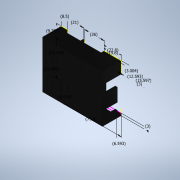
# Autodesk Inventor part: UNO Case
Saved by Autodesk Inventor 2020.1 (Build 241239000, 239)
## iProperties
Created: 2016-11-21
Part Number: UNO Case
Material: Generic
Document SubType Name: Modeling
Designer: Dimitris
Density: 1 g/cm^3
Appearance: Glossy - Black
Author: Dimitris
Autodesk Inventor part; units mm, degrees
ref_plane "YZ Plane" through (0, 0, 0) normal (1, 0, 0) x (0, 1, 0)
ref_plane "XZ Plane" through (0, 0, 0) normal (0, 1, 0) x (-1, 0, 0)
ref_plane "XY Plane" through (0, 0, 0) normal (0, 0, 1) x (1, 0, 0)
ref_plane "Work Plane2" through (0, 0, 0) normal (0, -1, 0) x (1, 0, 0)
sketch "Sketch33" plane through (0, 0, 0) normal (0, -1, 0) x (1, 0, 0)
  line L0 (74.8, -53.4338) -> (0, -53.4338)
  line L1 (0, -53.4338) -> (0, 0)
  line L2 (0, 0) -> (74.8, 0)
  line L3 (74.8, 0) -> (74.8, -53.4338)
  line L4 (74.8, -53.4338) -> (0, -53.4338)
  line L5 (0, -53.4338) -> (0, 0)
  line L6 (0, 0) -> (74.8, 0)
  line L7 (74.8, 0) -> (74.8, -53.4338)
  circle A0 centre (52, -49.5) radius 1.5 projected
  circle A1 centre (52, -49.5) radius 1.5
  circle A2 centre (3, -47.2929) radius 1.5 projected
  circle A3 centre (3, -47.2929) radius 1.5
  circle A4 centre (3, -15.7071) radius 1.5 projected
  circle A5 centre (3, -15.7071) radius 1.5
  circle A6 centre (55, -2.5) radius 1.5 projected
  circle A7 centre (55, -2.5) radius 1.5
  line L8 (74.8, -53.4338) -> (0, -53.4338)
  line L9 (0, -53.4338) -> (0, -58.4338)
  line L10 (0, -58.4338) -> (74.8, -58.4338)
  line L11 (74.8, -58.4338) -> (74.8, -53.4338)
  line L12 (0, -58.4338) -> (-5, -58.4338)
  line L13 (-5, -58.4338) -> (-5, -53.4338)
  line L14 (-5, -53.4338) -> (0, -53.4338)
  line L15 (0, -53.4338) -> (0, -58.4338)
  line L16 (0, 0) -> (-5, 0)
  line L17 (-5, 0) -> (-5, -53.4338)
  line L18 (-5, -53.4338) -> (0, -53.4338)
  line L19 (0, -53.4338) -> (0, 0)
  line L20 (-5, 0) -> (0, 0)
  line L21 (0, 0) -> (0, 5)
  line L22 (0, 5) -> (-5, 5)
  line L23 (-5, 5) -> (-5, 0)
  line L24 (0, 5) -> (74.8, 5)
  line L25 (74.8, 5) -> (74.8, 0)
  line L26 (74.8, 0) -> (0, 0)
  line L27 (0, 0) -> (0, 5)
  line L28 (74.8, -53.4338) -> (69.8, -53.4338)
  line L29 (69.8, -53.4338) -> (69.8, 5)
  line L30 (69.8, 5) -> (74.8, 5)
  line L31 (74.8, 5) -> (74.8, -53.4338)
  point P0 (74.8, 0)
  dimension "d220" = 5
  dimension "d221" = 5
  dimension "d222" = 5
  dimension "d223" = 5
  constraints: 64 end point, 16 parallel, 8 horizontal, 8 perpendicular, 4 centre point, 4 coincident, 3 point on line
  measures "d220" distance of L9.end L8.end
  measures "d221" distance of L13.end L14.end
  measures "d222" distance of L21.end L20.end
  measures "d223" distance of L29.end L30.end
extrude "Extrusion32" add sketch "Sketch33" along normal blind 5
ref_plane "Work Plane16" through (0, 0, 0) normal (0, 1, 0) x (1, 0, 0)
sketch "Sketch38" plane through (0, 0, 0) normal (0, 1, 0) x (1, 0, 0)
  line L0 (74.8, -5) -> (-5, -5) projected
  line L1 (-5, 58.4338) -> (74.8, 58.4338) projected
  line L2 (-5, -5) -> (-2, -5)
  line L3 (-2, -5) -> (-2, 58.4338)
  line L4 (-2, 58.4338) -> (-5, 58.4338)
  line L5 (-5, 58.4338) -> (-5, -5)
  line L6 (-5, -5) -> (-5, 58.4338) projected
  line L7 (74.8, 58.4338) -> (74.8, -5) projected
  line L8 (-5, 58.4338) -> (74.8, 58.4338)
  line L9 (74.8, 58.4338) -> (74.8, 55.4338)
  line L10 (74.8, 55.4338) -> (-5, 55.4338)
  line L11 (-5, 55.4338) -> (-5, 58.4338)
  line L12 (74.8, 58.4338) -> (71.8, 58.4338)
  line L13 (71.8, 58.4338) -> (71.8, 22.8825)
  line L14 (71.8, 22.8825) -> (74.8, 22.8825)
  line L15 (74.8, 22.8825) -> (74.8, 58.4338)
  line L16 (74.8, -5) -> (71.8, -5)
  line L17 (71.8, -5) -> (71.8, 10.5966)
  line L18 (71.8, 10.5966) -> (74.8, 10.5966)
  line L19 (74.8, 10.5966) -> (74.8, -5)
  line L20 (74.8, -5) -> (-5, -5)
  line L21 (-5, -5) -> (-5, -1.9965)
  line L22 (-5, -1.9965) -> (74.8, -1.9965)
  line L23 (74.8, -1.9965) -> (74.8, -5)
  point P0 (0, 0)
  point P1 (71.8, -1.9965)
  point P2 (-2, -1.9965)
  point P3 (-2, 55.4338)
  point P4 (71.8, 55.4338)
  dimension "d231" = 3
  dimension "d232" = 3
  dimension "d233" = 3
  constraints: 40 end point, 10 parallel, 6 point on line, 5 horizontal, 5 perpendicular
  measures "d231" distance of L4.end L3.end
  measures "d232" distance of L8.end L9.end
  measures "d233" distance of L14.end L13.end
extrude "Extrusion33" add sketch "Sketch38" along normal blind 20 contours L0 L17 L22 L7 | L0 L3 L22 L17 | L22 L17 L18 L7 | L0 L5 L22 L3 | L22 L5 L10 L3 | L14 L13 L10 L7 | L10 L5 L1 L3 | L3 L1 L13 L10 | L10 L13 L1 L7
ref_plane "Work Plane11" through (71.8, 0, 1.9965) normal (0, 0, -1) x (-1, 0, 0)
sketch "Sketch45" plane through (71.8, 0, 1.9965) normal (0, 0, -1) x (-1, 0, 0)
  line L0 (47.3, 2) -> (47.3, 11) projected
  line L1 (73.8, 0) -> (0, 0) projected
  line L2 (47.3, 11) -> (45.8, 11)
  line L3 (45.8, 11) -> (45.8, 0)
  line L4 (45.8, 0) -> (47.3, 0)
  line L5 (47.3, 0) -> (47.3, 11)
  line L6 (47.3, 11) -> (45.8, 11)
  line L7 (45.8, 11) -> (45.8, 20.3018)
  line L8 (45.8, 20.3018) -> (47.3, 20.3018)
  line L9 (47.3, 20.3018) -> (47.3, 11)
  line L10 (68.3, 11) -> (47.3, 11) projected
  line L11 (47.3, 20.3018) -> (68.3, 20.3018)
  line L12 (68.3, 20.3018) -> (68.3, 11)
  line L13 (68.3, 11) -> (47.3, 11)
  line L14 (47.3, 11) -> (47.3, 20.3018)
  line L15 (45.8, 11) -> (19.8, 11)
  line L16 (19.8, 11) -> (19.8, 20.3018)
  line L17 (19.8, 20.3018) -> (45.8, 20.3018)
  line L18 (45.8, 20.3018) -> (45.8, 11)
  point P0 (71.8, 0)
  dimension "d243" = 1.5
  dimension "d244" = 26
  constraints: 32 end point, 8 parallel, 4 horizontal, 4 perpendicular, 2 point on line
  measures "d243" distance of L4.end L3.end
  measures "d244" distance of L16.end L17.end
extrude "Extrusion37" cut sketch "Sketch45" against normal blind 10 contours L9 L11 L12 L10 | L15 L16 L17 L7
ref_plane "Work Plane10" through (0, 20, 0) normal (0, 1, 0) x (1, 0, 0)
sketch "Sketch46" plane through (0, 20, 0) normal (0, 1, 0) x (1, 0, 0)
  line L0 (-2, 55.4338) -> (71.8, 55.4338) projected
  line L1 (75.7583, 22.3753) -> (69.7041, 22.3753)
  line L2 (69.7041, 22.3753) -> (69.7041, 55.4338)
  line L3 (69.7041, 55.4338) -> (75.7583, 55.4338)
  line L4 (75.7583, 55.4338) -> (75.7583, 22.3753)
  point P0 (0, 0)
  constraints: 8 end point, 2 parallel, 1 horizontal, 1 perpendicular, 1 point on line
extrude "Extrusion38" cut sketch "Sketch46" against normal blind 5
ref_plane "Work Plane14" through (0, 15, 0) normal (0, 1, 0) x (1, 0, 0)
sketch "Sketch47" plane through (0, 15, 0) normal (0, 1, 0) x (1, 0, 0)
  line L0 (70.1, 40.5) -> (70.1, 49.5) projected
  line L1 (70.1, 40.5) -> (76.1155, 40.5)
  line L2 (76.1155, 40.5) -> (76.1155, 49.5)
  line L3 (76.1155, 49.5) -> (70.1, 49.5)
  line L4 (70.1, 49.5) -> (70.1, 40.5)
  point P0 (0, 0)
  dimension "d249" = 9
  constraints: 8 end point, 2 parallel, 1 horizontal, 1 perpendicular
  measures "d249" distance of L2.end L1.end
extrude "Extrusion39" cut sketch "Sketch47" against normal blind 15
ref_plane "Work Plane9" through (0, 20, 0) normal (0, 1, 0) x (1, 0, 0)
sketch "Sketch48" plane through (0, 20, 0) normal (0, 1, 0) x (1, 0, 0)
  line L0 (74.8, 58.4338) -> (-5, 58.4338) projected
  line L1 (68.5228, 52.4259) -> (68.2069, 52.4259)
  line L2 (68.2069, 52.4259) -> (68.2069, 58.4338)
  line L3 (68.2069, 58.4338) -> (68.5228, 58.4338)
  line L4 (68.5228, 58.4338) -> (68.5228, 52.4259)
  line L5 (68.2069, 58.4338) -> (68.5228, 58.4338)
  line L6 (68.5228, 58.4338) -> (68.5228, 53.4262)
  line L7 (68.5228, 53.4262) -> (68.2069, 53.4262)
  line L8 (68.2069, 53.4262) -> (68.2069, 58.4338)
  line L9 (-2, 55.4338) -> (74.8, 55.4338) projected
  line L10 (68.5228, 55.4338) -> (50.5228, 55.4338)
  line L11 (50.5228, 55.4338) -> (50.5228, 58.4338)
  line L12 (50.5228, 58.4338) -> (68.5228, 58.4338)
  line L13 (68.5228, 58.4338) -> (68.5228, 55.4338)
  line L14 (51.9394, 55.4338) -> (3.9394, 55.4338)
  line L15 (3.9394, 55.4338) -> (3.9394, 58.4338)
  line L16 (3.9394, 58.4338) -> (51.9394, 58.4338)
  line L17 (51.9394, 58.4338) -> (51.9394, 55.4338)
  line L18 (-5, 58.4338) -> (-5, -5) projected
  line L19 (-5, 44.9754) -> (3.9394, 44.9754)
  line L20 (3.9394, 44.9754) -> (3.9394, 17.8349)
  line L21 (3.9394, 17.8349) -> (-5, 17.8349)
  line L22 (-5, 17.8349) -> (-5, 44.9754)
  line L23 (-5, 12.2802) -> (-0.5303, 12.2802)
  line L24 (-0.5303, 12.2802) -> (-0.5303, 2.9287)
  line L25 (-0.5303, 2.9287) -> (-5, 2.9287)
  line L26 (-5, 2.9287) -> (-5, 12.2802)
  point P0 (0, 0)
  point P1 (68.2069, 55.4338)
  dimension "d252" = 18
  dimension "d253" = 48
  constraints: 48 end point, 12 parallel, 10 point on line, 6 horizontal, 6 perpendicular
  measures "d252" distance of L11.end L12.end
  measures "d253" distance of L15.end L16.end
ref_plane "Work Plane8" through (0, 20, 0) normal (0, 1, 0) x (1, 0, 0)
sketch "Sketch49" plane through (0, 20, 0) normal (0, 1, 0) x (1, 0, 0)
  line L0 (74.8, 58.4338) -> (-5, 58.4338) projected
  line L1 (-2, 55.4338) -> (74.8, 55.4338) projected
  line L2 (50.5217, 58.4338) -> (3.9392, 58.4338)
  line L3 (3.9392, 58.4338) -> (3.9392, 55.4338)
  line L4 (3.9392, 55.4338) -> (50.5217, 55.4338)
  line L5 (50.5217, 55.4338) -> (50.5217, 58.4338)
  point P0 (0, 0)
  constraints: 8 end point, 2 parallel, 2 point on line, 1 horizontal, 1 perpendicular
extrude "Extrusion40" cut sketch "Sketch48" against normal blind 5 contours L23 L24 L25 L18 | L19 L20 L21 L18 | L2 L9 L17 L0 | L17 L9 L11 L0 | L11 L9 L15 L0
ref_plane "Work Plane13" through (26, 11, 1.9965) normal (0, 1, 0) x (1, 0, 0)
sketch "Sketch50" plane through (26, 11, 1.9965) normal (0, 1, 0) x (1, 0, 0)
  line L0 (-1.5, 0) -> (-1.5, -3.0035) projected
  line L1 (-31, -3.0035) -> (-22.5, -3.0035) projected
  line L2 (-1.5, 0) -> (-22.5, 0)
  line L3 (-22.5, 0) -> (-22.5, -3.0035)
  line L4 (-22.5, -3.0035) -> (-1.5, -3.0035)
  line L5 (-1.5, -3.0035) -> (-1.5, 0)
  line L6 (0, 0) -> (0, -3.0035) projected
  line L7 (26, 0) -> (26, -3.0035) projected
  line L8 (0, -3.0035) -> (26, -3.0035)
  line L9 (26, -3.0035) -> (26, 0)
  line L10 (26, 0) -> (0, 0)
  line L11 (0, 0) -> (0, -3.0035)
  point P0 (-26, 1.9965)
  point P1 (26, -3.0035)
  constraints: 16 end point, 4 parallel, 2 horizontal, 2 perpendicular
extrude "Extrusion41" add sketch "Sketch50" along normal blind 5
sketch "Sketch51" plane through (0, 20, 0) normal (0, 1, 0) x (1, 0, 0)
  point P0 (0, 0)
sketch "Sketch52" plane through (0, 20, 0) normal (0, 1, 0) x (1, 0, 0)
  line L0 (3.9394, 58.4338) -> (-5, 58.4338) projected
  line L1 (-5, -5) -> (3.5, -5) projected
  line L2 (74.8, 55.4338) -> (74.8, 49.5) projected
  line L3 (-5, 58.4338) -> (-5, 44.9754) projected
  line L4 (74.8, 55.4338) -> (74.8, 58.4338) projected
  line L5 (68.2069, 58.4338) -> (68.2069, 55.4338) projected
  line L6 (74.8, -5) -> (74.8, 10.5966) projected
  line L7 (52, -1.9965) -> (52, -5) projected
  line L8 (52, -5) -> (74.8, -5) projected
  line L9 (71.8, -1.9965) -> (52, -1.9965) projected
  line L10 (71.8, 10.5966) -> (71.8, -1.9965) projected
  line L11 (26, -5) -> (26, -1.9965) projected
  line L12 (24.5, -1.9965) -> (24.5, -5) projected
  line L13 (3.5, -5) -> (3.5, -1.9965) projected
  line L14 (-5, 12.2802) -> (-2, 12.2802) projected
  line L15 (-2, 2.9287) -> (-5, 2.9287) projected
  point P0 (0, 0)
  dimension "d258" = 63.4338
  dimension "d259" = 79.8
  dimension "d260" = 6.5931
  dimension "d261" = 3
  dimension "d262" = 22.8
  dimension "d263" = 3.0035
  dimension "d264" = 3
  dimension "d265" = 12.593
  dimension "d266" = 15.5966
  dimension "d267" = 19.8
  dimension "d268" = 26
  dimension "d269" = 21
  dimension "d270" = 8.5
  dimension "d271" = 9.3515
  dimension "d272" = 13.4584
  dimension "d273" = 8.9394
  measures "d258" distance between parallel lines of L0 L1
  measures "d259" distance between parallel lines of L2 L3
  measures "d260" distance between parallel lines of L4 L5
  measures "d261" distance of L2.start L4.end
  measures "d262" distance between parallel lines of L6 L7
  measures "d263" distance between parallel lines of L8 L9
  measures "d264" distance between parallel lines of L6 L10
  measures "d265" distance of L10.start L9.start
  measures "d266" distance of L6.start L6.end
  measures "d267" distance of L9.start L7.start
  measures "d268" distance between parallel lines of L7 L11
  measures "d269" distance between parallel lines of L12 L13
  measures "d270" distance of L1.start L1.end
  measures "d271" distance between parallel lines of L14 L15
  measures "d272" distance of L0.end L3.end
  measures "d273" distance of L0.start L0.end
body "Solid1"
